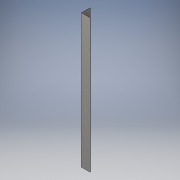
# Autodesk Inventor part: 24-inch-L
Saved by Autodesk Inventor 2017 (Build 210142000, 142)
## iProperties
Created: 2017-08-30
Part Number: 24-inch-L
Material: Generic
Document SubType Name: Modeling
Designer: Trent
Density: 1 g/cm^3
Appearance: Default
Author: Trent
Autodesk Inventor part; units mm, degrees
ref_plane "YZ Plane" through (0, 0, 0) normal (1, 0, 0) x (0, 1, 0)
ref_plane "XZ Plane" through (0, 0, 0) normal (0, 1, 0) x (-1, 0, 0)
ref_plane "XY Plane" through (0, 0, 0) normal (0, 0, 1) x (1, 0, 0)
sketch "Sketch1" plane through (0, 0, 0) normal (0, 1, 0) x (-1, 0, 0)
  line L0 (0, 0) -> (0, -38.1)
  line L1 (0, 0) -> (-38.1, 0)
  line L2 (1.5875, -38.1) -> (1.5875, 1.5875)
  line L3 (1.5875, 1.5875) -> (-38.1, 1.5875)
  line L4 (1.5875, -38.1) -> (0, -38.1)
  line L5 (-38.1, 1.5875) -> (-38.1, 0)
  dimension "d0" = 38.1
  dimension "d1" = 38.1
  dimension "d2" = 1.5875
  constraints: 12 end point, 2 horizontal, 1 perpendicular, 1 vertical, 1 other
  measures "d0" distance of L0.start L0.end
  measures "d1" distance of L0.start L1.end
  measures "d2" distance between parallel lines of L0 L2
extrude "Extrusion1" add sketch "Sketch1" along normal blind 609.6
body "Solid1"
